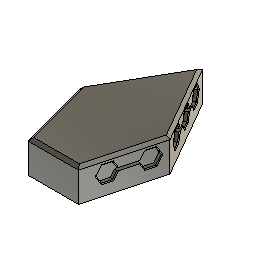
wedge_30deg_0mm (Autodesk Fusion 360 design; units mm, degrees)
Autodesk Fusion 360 part; units mm, degrees
note: some values were not read from the file. Set by a fixed rule: which sketch regions a step uses.
sketch "case_bottom" plane through (0, 0, 0) normal (0, 0, 1) x (1, 0, 0)
  line L0 (-89.0663, -56.676) -> (12.947, -115.5733)
  line L1 (-48.1807, 14.1399) -> (-89.0663, -56.676)
  line L2 (12.947, -115.5733) -> (30.0588, -101.2149)
  line L3 (-25.0151, 15.0605) -> (-48.1807, 14.1399)
  line L4 (11.7937, -0.3589) -> (11.7217, -0.2966)
  line L5 (11.7217, -0.2966) -> (-4.9219, 9.3126)
  line L6 (42.4432, -26.8948) -> (11.7937, -0.3589)
  line L7 (30.0588, -101.2149) -> (20.3625, -65.1396)
  line L8 (20.3625, -65.1396) -> (42.4432, -26.8948)
  line L9 (-4.9219, 9.3126) -> (-25.0151, 15.0605)
  line L10 (-49.952, 17.0719) -> (-93.1644, -57.774)
  line L11 (-93.1644, -57.774) -> (13.2662, -119.2217)
  line L12 (13.4693, 2.1586) -> (-3.7417, 12.0954)
  line L13 (-3.7417, 12.0954) -> (-24.653, 18.0773)
  line L14 (13.2662, -119.2217) -> (33.4524, -102.2834)
  line L15 (23.5826, -65.5623) -> (46.2803, -26.2487)
  line L16 (33.4524, -102.2834) -> (23.5826, -65.5623)
  line L17 (-24.653, 18.0773) -> (-49.952, 17.0719)
  line L18 (46.2803, -26.2487) -> (13.4693, 2.1586)
  line L19 (-4.4498, 10.4257) -> (-24.8703, 16.2672)
  line L20 (-48.8893, 15.3127) -> (-90.7055, -57.1152)
  line L21 (43.9781, -26.6364) -> (12.4207, 0.6855)
  line L22 (13.0747, -117.0327) -> (31.4162, -101.6423)
  line L23 (12.4207, 0.6855) -> (-4.4498, 10.4257)
  line L24 (-24.8703, 16.2672) -> (-48.8893, 15.3127)
  line L25 (31.4162, -101.6423) -> (21.6506, -65.3087)
  line L26 (21.6506, -65.3087) -> (43.9781, -26.6364)
  line L27 (-90.7055, -57.1152) -> (13.0747, -117.0327)
  line L28 (-4.2138, 10.9823) -> (-24.7979, 16.8706)
  line L29 (-91.5252, -57.3348) -> (13.1385, -117.7624)
  line L30 (-49.2435, 15.8991) -> (-91.5252, -57.3348)
  line L31 (12.9719, 1.0019) -> (12.7702, 1.1765)
  line L32 (32.095, -101.856) -> (22.2946, -65.3932)
  line L33 (22.2946, -65.3932) -> (44.7455, -26.5072)
  line L34 (13.1385, -117.7624) -> (32.095, -101.856)
  line L35 (12.7702, 1.1765) -> (-4.2138, 10.9823)
  line L36 (-24.7979, 16.8706) -> (-49.2435, 15.8991)
  line L37 (44.7455, -26.5072) -> (12.9719, 1.0019)
  circle A0 centre (-32.1047, -5.0156) radius 2.2
  circle A1 centre (-51.1047, -37.9246) radius 2.2
  circle A2 centre (12.9286, -31.0156) radius 2.2
  circle A3 centre (4.9904, -77.0362) radius 2.2
  line L38 (-48.2004, -55.8942) -> (-76.7793, -39.3942)
  line L39 (-57.2004, -71.4826) -> (-48.2004, -55.8942)
  line L40 (-85.7793, -54.9826) -> (-57.2004, -71.4826)
  line L41 (-76.7793, -39.3942) -> (-85.7793, -54.9826)
  line L42 (-52.8377, -70.9761) -> (-55.7627, -76.0424)
  line L43 (-48.1417, -80.4424) -> (-45.2167, -75.3761)
  line L44 (-45.2167, -75.3761) -> (-52.8377, -70.9761)
  line L45 (-37.9329, -84.7603) -> (-36.1829, -81.7292)
  line L46 (-43.9771, -77.2292) -> (-45.7271, -80.2603)
  line L47 (-45.7271, -80.2603) -> (-37.9329, -84.7603)
  line L48 (-36.1829, -81.7292) -> (-43.9771, -77.2292)
  line L49 (25.0269, -87.2736) -> (22.1799, -76.6484)
  line L50 (16.237, -89.6289) -> (25.0269, -87.2736)
  line L51 (13.3899, -79.0037) -> (16.237, -89.6289)
  line L52 (22.1799, -76.6484) -> (13.3899, -79.0037)
  line L53 (-49.878, -40.9999) -> (-54.328, -48.7075)
  line L54 (-54.328, -48.7075) -> (-46.8802, -53.0075)
  line L55 (-46.8802, -53.0075) -> (-42.4302, -45.2999)
  line L56 (-42.4302, -45.2999) -> (-49.878, -40.9999)
  line L57 (46.2803, -26.2487) -> (46.2803, -130.4054) construction
  line L58 (178.3399, -54.9826) -> (149.761, -71.4826)
  line L59 (140.7023, -80.4424) -> (137.7773, -75.3761)
  line L60 (70.266, -65.3932) -> (47.8152, -26.5072)
  line L61 (80.7669, -0.3589) -> (80.8389, -0.2966)
  line L62 (145.3983, -70.9761) -> (148.3233, -76.0424)
  circle A4 centre (87.5702, -77.0362) radius 2.2
  line L63 (137.7773, -75.3761) -> (145.3983, -70.9761)
  line L64 (136.5377, -77.2292) -> (138.2877, -80.2603)
  line L65 (128.7435, -81.7292) -> (136.5377, -77.2292)
  line L66 (76.3237, -89.6289) -> (67.5338, -87.2736)
  line L67 (62.5019, -101.2149) -> (72.1981, -65.1396)
  line L68 (79.2945, -119.2217) -> (59.1082, -102.2834)
  line L69 (79.486, -117.0327) -> (61.1444, -101.6423)
  line L70 (70.3808, -76.6484) -> (79.1707, -79.0037)
  line L71 (142.4387, -40.9999) -> (146.8887, -48.7075)
  line L72 (130.4935, -84.7603) -> (128.7435, -81.7292)
  line L73 (67.5338, -87.2736) -> (70.3808, -76.6484)
  line L74 (138.2877, -80.2603) -> (130.4935, -84.7603)
  line L75 (142.5127, 17.0719) -> (185.725, -57.774)
  line L76 (80.1399, 0.6855) -> (97.0105, 10.4257)
  line L77 (48.5826, -26.6364) -> (80.1399, 0.6855)
  line L78 (46.2803, -26.2487) -> (79.0914, 2.1586)
  line L79 (117.2137, 18.0773) -> (142.5127, 17.0719)
  line L80 (79.0914, 2.1586) -> (96.3024, 12.0954)
  line L81 (97.4825, 9.3126) -> (117.5757, 15.0605)
  circle A5 centre (124.6653, -5.0156) radius 2.2
  line L82 (134.9909, -45.2999) -> (142.4387, -40.9999)
  line L83 (169.3399, -39.3942) -> (178.3399, -54.9826)
  line L84 (139.4409, -53.0075) -> (134.9909, -45.2999)
  line L85 (117.3585, 16.8706) -> (141.8041, 15.8991)
  line L86 (146.8887, -48.7075) -> (139.4409, -53.0075)
  line L87 (79.5887, 1.0019) -> (79.7904, 1.1765)
  line L88 (50.1174, -26.8948) -> (80.7669, -0.3589)
  line L89 (149.761, -71.4826) -> (140.761, -55.8942)
  line L90 (184.0858, -57.3348) -> (79.4221, -117.7624)
  line L91 (60.4657, -101.856) -> (70.266, -65.3932)
  line L92 (79.6136, -115.5733) -> (62.5019, -101.2149)
  line L93 (183.2662, -57.1152) -> (79.486, -117.0327)
  line L94 (79.4221, -117.7624) -> (60.4657, -101.856)
  line L95 (47.8152, -26.5072) -> (79.5887, 1.0019)
  line L96 (141.4499, 15.3127) -> (183.2662, -57.1152)
  line L97 (80.8389, -0.2966) -> (97.4825, 9.3126)
  circle A6 centre (143.6653, -37.9246) radius 2.2
  line L98 (140.761, -55.8942) -> (169.3399, -39.3942)
  line L99 (61.1444, -101.6423) -> (70.9101, -65.3087)
  line L100 (59.1082, -102.2834) -> (68.978, -65.5623)
  line L101 (79.1707, -79.0037) -> (76.3237, -89.6289)
  line L102 (185.725, -57.774) -> (79.2945, -119.2217)
  line L103 (181.6269, -56.676) -> (79.6136, -115.5733)
  line L104 (140.7414, 14.1399) -> (181.6269, -56.676)
  line L105 (96.7744, 10.9823) -> (117.3585, 16.8706)
  line L106 (79.7904, 1.1765) -> (96.7744, 10.9823)
  line L107 (96.3024, 12.0954) -> (117.2137, 18.0773)
  line L108 (70.9101, -65.3087) -> (48.5826, -26.6364)
  line L109 (97.0105, 10.4257) -> (117.4309, 16.2672)
  line L110 (117.4309, 16.2672) -> (141.4499, 15.3127)
  line L111 (141.8041, 15.8991) -> (184.0858, -57.3348)
  line L112 (117.5757, 15.0605) -> (140.7414, 14.1399)
  circle A7 centre (79.632, -31.0156) radius 2.2
  line L113 (72.1981, -65.1396) -> (50.1174, -26.8948)
  line L114 (68.978, -65.5623) -> (46.2803, -26.2487)
  line L115 (33.4524, -102.2834) -> (59.1082, -102.2834)
  dimension "d81" = 1.5
  constraint vertical L57
  constraint horizontal L115
extrude "Extrude2" add sketch "case_bottom" along normal blind 16.6 contours L15 L16 L100 L114 L115
sketch "Sketch13" plane through (23.3442, 13.4778, 0) normal (0.866025, 0.5, 0) x (-0.5, 0.866025, 0)
  line L0 (-91.2676, 0) -> (-45.8722, 0)
  line L1 (-45.8722, 0) -> (-45.8722, 16.6)
  line L2 (-45.8722, 16.6) -> (-91.2676, 16.6)
  line L3 (-91.2676, 16.6) -> (-91.2676, 0)
  line L4 (-91.2676, 9.7) -> (-45.8722, 9.7) construction
  line L5 (-79.2676, 13.6708) -> (-83.8576, 13.6792)
  line L6 (-83.8576, 13.6792) -> (-86.1599, 9.7085)
  line L7 (-86.1599, 9.7085) -> (-83.8722, 5.7292)
  line L8 (-83.8722, 5.7292) -> (-79.2823, 5.7208)
  line L9 (-79.2823, 5.7208) -> (-76.98, 9.6915)
  line L10 (-76.98, 9.6915) -> (-79.2676, 13.6708)
  line L11 (-66.2676, 13.6708) -> (-70.8576, 13.6792)
  line L12 (-70.8576, 13.6792) -> (-73.1599, 9.7085)
  line L13 (-73.1599, 9.7085) -> (-70.8722, 5.7292)
  line L14 (-70.8722, 5.7292) -> (-66.2823, 5.7208)
  line L15 (-66.2823, 5.7208) -> (-63.98, 9.6915)
  line L16 (-63.98, 9.6915) -> (-66.2676, 13.6708)
  line L17 (-53.2676, 13.6708) -> (-57.8576, 13.6792)
  line L18 (-57.8576, 13.6792) -> (-60.1599, 9.7085)
  line L19 (-60.1599, 9.7085) -> (-57.8722, 5.7292)
  line L20 (-57.8722, 5.7292) -> (-53.2823, 5.7208)
  line L21 (-53.2823, 5.7208) -> (-50.98, 9.6915)
  line L22 (-50.98, 9.6915) -> (-53.2676, 13.6708)
  line L23 (-81.5699, 8.95) -> (-55.5699, 8.95)
  arc A0 (-55.5699, 8.95) -> (-55.5699, 10.45) centre (-55.5699, 9.7) ccw
  line L24 (-55.5699, 10.45) -> (-81.5699, 10.45)
  arc A1 (-81.5699, 10.45) -> (-81.5699, 8.95) centre (-81.5699, 9.7) ccw
  line L25 (-81.5699, 9.7) -> (-55.5699, 9.7) construction
  point P0 (-68.5699, 9.7)
  point P1 (-81.5699, 9.7)
  point P2 (-55.5699, 9.7)
  point P3 (-81.5699, 9.7)
  point P4 (-68.5699, 9.7)
  point P5 (-55.5699, 9.7)
  dimension "d99" = 6.9
  dimension "d100" = 13
  dimension "d101" = 13
  dimension "d102" = 3.975
  dimension "d103" = 3.975
  dimension "d104" = 3.975
  dimension "d105" = 1.5
  constraint coincident L3 L4.start
  constraint coincident L1 L4.end
  constraint perpendicular L1 L4
  constraint midpoint L4 P4
  constraint coincident L4 P3
  constraint coincident L4 P5
  constraint coincident P3 P1
  constraint coincident P4 P0
  constraint coincident P5 P2
  constraint tangent L23 A0
  constraint tangent A0 L24
  constraint parallel L23 L24
  constraint tangent L24 A1
  constraint tangent L23 A1
  constraint parallel L4 L25
  measures "d99" distance of L2 L4
  measures "d100" distance of P4 P5
  measures "d101" distance of P4 P3
  measures "d102" distance of P3 L10
  measures "d103" distance of P4 L16
  measures "d104" distance of P5 L22
  measures "d105" diameter of A0
extrude "Extrude15" cut sketch "Sketch13" against normal blind 2 contours L5 L6 L7 L8 L9 L10 L23 L24 A1 | L9 L10 L12 L13 L23 L24 | L9 L10 L23 L24 A1 | L12 L13 L15 L16 L23 L24 | L11 L12 L16 L24 | L15 L16 L18 L19 L23 L24 | L13 L14 L15 L23 | L18 L19 L23 A0 L24 | L17 L18 L19 L20 L21 L22 L23 A0 L24
sketch "Sketch14" plane through (46.0763, -26.6022, 0) normal (-0.866025, 0.5, 0) x (-0.5, -0.866025, 0)
  line L0 (-0.4081, 0) -> (44.9873, 0)
  line L1 (44.9873, 0) -> (44.9873, 16.6)
  line L2 (44.9873, 16.6) -> (-0.4081, 16.6)
  line L3 (-0.4081, 16.6) -> (-0.4081, 0)
  line L4 (-0.4081, 9.7) -> (44.9873, 9.7) construction
  line L5 (11.5797, 13.6778) -> (6.9897, 13.6722)
  line L6 (6.9897, 13.6722) -> (4.6997, 9.6943)
  line L7 (4.6997, 9.6943) -> (6.9996, 5.7222)
  line L8 (6.9996, 5.7222) -> (11.5895, 5.7278)
  line L9 (11.5895, 5.7278) -> (13.8795, 9.7057)
  line L10 (13.8795, 9.7057) -> (11.5797, 13.6778)
  line L11 (24.5797, 13.6778) -> (19.9897, 13.6722)
  line L12 (19.9897, 13.6722) -> (17.6997, 9.6943)
  line L13 (17.6997, 9.6943) -> (19.9996, 5.7222)
  line L14 (19.9996, 5.7222) -> (24.5895, 5.7278)
  line L15 (24.5895, 5.7278) -> (26.8795, 9.7057)
  line L16 (26.8795, 9.7057) -> (24.5797, 13.6778)
  line L17 (37.5797, 13.6778) -> (32.9897, 13.6722)
  line L18 (32.9897, 13.6722) -> (30.6997, 9.6943)
  line L19 (30.6997, 9.6943) -> (32.9996, 5.7222)
  line L20 (32.9996, 5.7222) -> (37.5895, 5.7278)
  line L21 (37.5895, 5.7278) -> (39.8795, 9.7057)
  line L22 (39.8795, 9.7057) -> (37.5797, 13.6778)
  line L23 (9.2896, 8.95) -> (35.2896, 8.95)
  arc A0 (35.2896, 8.95) -> (35.2896, 10.45) centre (35.2896, 9.7) ccw
  line L24 (35.2896, 10.45) -> (9.2896, 10.45)
  arc A1 (9.2896, 10.45) -> (9.2896, 8.95) centre (9.2896, 9.7) ccw
  line L25 (9.2896, 9.7) -> (35.2896, 9.7) construction
  point P0 (22.2896, 9.7)
  point P1 (35.2896, 9.7)
  point P2 (9.2896, 9.7)
  point P3 (9.2896, 9.7)
  point P4 (22.2896, 9.7)
  point P5 (35.2896, 9.7)
  dimension "d108" = 6.9
  dimension "d109" = 13
  dimension "d110" = 13
  dimension "d111" = 3.975
  dimension "d112" = 3.975
  dimension "d113" = 3.975
  dimension "d114" = 1.5
  constraint coincident L3 L4.start
  constraint coincident L1 L4.end
  constraint perpendicular L1 L4
  constraint midpoint L4 P4
  constraint coincident L4 P5
  constraint coincident L4 P3
  constraint coincident P3 P2
  constraint coincident P4 P0
  constraint coincident P5 P1
  constraint tangent L23 A0
  constraint tangent A0 L24
  constraint parallel L23 L24
  constraint tangent L24 A1
  constraint tangent L23 A1
  constraint parallel L4 L25
  measures "d108" distance of L2 L4
  measures "d109" distance of P4 P3
  measures "d110" distance of P4 P5
  measures "d111" distance of P3 L10
  measures "d112" distance of P4 L16
  measures "d113" distance of P5 L22
  measures "d114" diameter of A0
extrude "Extrude16" cut sketch "Sketch14" against normal blind 2 contours L5 L6 L7 L8 L9 L10 L23 L24 A1 | L9 L10 L12 L13 L23 L24 | L9 L10 L23 L24 A1 | L12 L13 L15 L16 L23 L24 | L11 L12 L16 L24 | L15 L16 L18 L19 L23 L24 | L13 L14 L15 L23 | L18 L19 L23 A0 L24 | L17 L18 L19 L20 L21 L22 L23 A0 L24
sketch "Sketch15" plane through (5.5593, 1.4942, 0) normal (-0.965726, -0.259565, 0) x (0.259565, -0.965726, 0)
  line L0 (69.4364, 0) -> (107.4608, 0)
  line L1 (107.4608, 0) -> (107.4608, 16.6)
  line L2 (107.4608, 16.6) -> (69.4364, 16.6)
  line L3 (69.4364, 16.6) -> (69.4364, 0)
  line L4 (69.4364, 9.7) -> (107.4608, 9.7) construction
  line L5 (79.7376, 13.6714) -> (75.1477, 13.6786)
  line L6 (75.1477, 13.6786) -> (72.8465, 9.7072)
  line L7 (72.8465, 9.7072) -> (75.1352, 5.7286)
  line L8 (75.1352, 5.7286) -> (79.7251, 5.7214)
  line L9 (79.7251, 5.7214) -> (82.0264, 9.6928)
  line L10 (82.0264, 9.6928) -> (79.7376, 13.6714)
  line L11 (90.8709, 9.6928) -> (93.1721, 5.7214)
  line L12 (93.1721, 5.7214) -> (97.762, 5.7286)
  line L13 (97.762, 5.7286) -> (100.0508, 9.7072)
  line L14 (100.0508, 9.7072) -> (97.7495, 13.6786)
  line L15 (97.7495, 13.6786) -> (93.1596, 13.6714)
  line L16 (93.1596, 13.6714) -> (90.8709, 9.6928)
  line L17 (77.4364, 8.95) -> (95.4608, 8.95)
  arc A0 (95.4608, 8.95) -> (95.4608, 10.45) centre (95.4608, 9.7) ccw
  line L18 (95.4608, 10.45) -> (77.4364, 10.45)
  arc A1 (77.4364, 10.45) -> (77.4364, 8.95) centre (77.4364, 9.7) ccw
  line L19 (77.4364, 9.7) -> (95.4608, 9.7) construction
  point P0 (77.4364, 9.7)
  point P1 (95.4608, 9.7)
  point P2 (77.4364, 9.7)
  point P3 (95.4608, 9.7)
  dimension "d117" = 6.9
  dimension "d118" = 8
  dimension "d119" = 12
  dimension "d120" = 3.975
  dimension "d121" = 3.975
  dimension "d122" = 1.5
  constraint coincident L3 L4.start
  constraint coincident L1 L4.end
  constraint perpendicular L1 L4
  constraint coincident L4 P2
  constraint coincident L4 P3
  constraint coincident P2 P0
  constraint coincident P3 P1
  constraint tangent L17 A0
  constraint tangent A0 L18
  constraint parallel L17 L18
  constraint tangent L18 A1
  constraint tangent L17 A1
  constraint parallel L4 L19
  measures "d117" distance of L2 L4
  measures "d118" distance of L3 P2
  measures "d119" distance of L1 P3
  measures "d120" distance of P2 L10
  measures "d121" distance of P3 L16
  measures "d122" diameter of A0
extrude "Extrude17" cut sketch "Sketch15" against normal blind 2 contours L5 L6 L7 L8 L9 L10 L17 L18 A1 | L9 L10 L11 L16 L17 L18 | L9 L10 L17 L18 A1 | L11 L16 L17 A0 L18 | L11 L12 L13 L14 L15 L16 L17 A0 L18
sketch "Sketch16" plane through (80.7651, -21.7078, 0) normal (0.965726, -0.259565, 0) x (0.259565, 0.965726, 0)
  line L0 (-83.4353, 0) -> (-45.4109, 0)
  line L1 (-45.4109, 0) -> (-45.4109, 16.6)
  line L2 (-45.4109, 16.6) -> (-83.4353, 16.6)
  line L3 (-83.4353, 16.6) -> (-83.4353, 0)
  line L4 (-83.4353, 9.7) -> (-45.4109, 9.7) construction
  line L5 (-69.1608, 13.6868) -> (-73.7507, 13.6631)
  line L6 (-73.7507, 13.6631) -> (-76.0252, 9.6764)
  line L7 (-76.0252, 9.6764) -> (-73.7098, 5.7132)
  line L8 (-73.7098, 5.7132) -> (-69.1199, 5.7369)
  line L9 (-69.1199, 5.7369) -> (-66.8454, 9.7236)
  line L10 (-66.8454, 9.7236) -> (-69.1608, 13.6868)
  line L11 (-58.0008, 9.7236) -> (-55.7263, 5.7369)
  line L12 (-55.7263, 5.7369) -> (-51.1364, 5.7132)
  line L13 (-51.1364, 5.7132) -> (-48.821, 9.6764)
  line L14 (-48.821, 9.6764) -> (-51.0955, 13.6631)
  line L15 (-51.0955, 13.6631) -> (-55.6854, 13.6868)
  line L16 (-55.6854, 13.6868) -> (-58.0008, 9.7236)
  line L17 (-53.4109, 10.45) -> (-71.4353, 10.45)
  arc A0 (-71.4353, 10.45) -> (-71.4353, 8.95) centre (-71.4353, 9.7) ccw
  line L18 (-71.4353, 8.95) -> (-53.4109, 8.95)
  arc A1 (-53.4109, 8.95) -> (-53.4109, 10.45) centre (-53.4109, 9.7) ccw
  line L19 (-53.4109, 9.7) -> (-71.4353, 9.7) construction
  point P0 (-71.4353, 9.7)
  point P1 (-53.4109, 9.7)
  point P2 (-71.4353, 9.7)
  point P3 (-53.4109, 9.7)
  dimension "d125" = 6.9
  dimension "d126" = 8
  dimension "d127" = 12
  dimension "d128" = 3.975
  dimension "d129" = 3.975
  dimension "d130" = 1.5
  constraint coincident L3 L4.start
  constraint coincident L1 L4.end
  constraint perpendicular L1 L4
  constraint coincident L4 P2
  constraint coincident L4 P3
  constraint coincident P2 P0
  constraint coincident P3 P1
  constraint tangent L17 A0
  constraint tangent A0 L18
  constraint parallel L17 L18
  constraint tangent L18 A1
  constraint tangent L17 A1
  constraint parallel L4 L19
  measures "d125" distance of L2 L4
  measures "d126" distance of L1 P3
  measures "d127" distance of L3 P2
  measures "d128" distance of P2 L10
  measures "d129" distance of P3 L16
  measures "d130" diameter of A0
extrude "Extrude18" cut sketch "Sketch16" against normal blind 2 contours L5 L6 L7 L8 L9 L10 L17 A0 L18 | L9 L10 L11 L16 L17 L18 | L9 L10 L17 A0 L18 | L11 L16 L17 L18 A1 | L11 L12 L13 L14 L15 L16 L17 L18 A1
chamfer "Chamfer4" distance 0.4 angle 45 60 edges at (43.1539, -31.6638, 11.6832) (41.4339, -34.6429, 13.675) (43.1515, -31.6681, 7.7082) (41.429, -34.6514, 5.725) (39.8178, -37.4422, 7.3389) (39.8192, -37.4397, 12.0639) (36.5452, -43.1105, 12.0611) (34.9339, -45.9013, 13.675) (33.3192, -48.698, 12.0639) (36.5437, -43.113, 7.3361) (34.929, -45.9098, 5.725) (33.3178, -48.7005, 7.3389) (30.0452, -54.3689, 12.0611) (28.4339, -57.1596, 13.675) (26.7115, -60.143, 11.6918) (26.709, -60.1472, 7.7168) (28.429, -57.1681, 5.725) (30.0437, -54.3713, 7.3361) (24.7664, -69.9667, 11.6929) (25.6608, -73.2942, 13.675) (26.497, -76.4053, 12.0607) (24.7648, -69.9606, 7.7179) (25.6575, -73.2821, 5.725) (26.496, -76.4017, 7.3357) (29.4998, -87.5776, 12.0607) (30.336, -90.6887, 13.675) (29.5008, -87.5811, 7.3357) (30.3393, -90.7008, 5.725) (31.232, -94.0222, 7.7179) (31.2304, -94.0162, 11.6929) (62.2177, -90.7145, 13.6749) (61.3268, -94.029, 11.6697) (61.3321, -94.0093, 7.6948) (62.2283, -90.675, 5.7251) (63.0619, -87.5736, 7.3434) (63.0588, -87.5851, 12.0684) (66.0657, -76.3977, 12.0684) (66.9068, -73.2683, 13.6749) (66.0626, -76.4093, 7.3434) (66.8962, -73.3079, 5.7251) (67.7924, -69.9736, 7.6948) (67.7977, -69.9538, 11.6697) (65.8486, -60.1419, 11.6939) (65.8522, -60.1483, 7.7189) (64.1255, -57.1575, 13.675) (62.5151, -54.3682, 12.0604) (64.1328, -57.1702, 5.725) (62.5173, -54.372, 7.3354) (59.2411, -48.6974, 12.0646) (59.2432, -48.7011, 7.3396) (57.6328, -45.9119, 5.725) (56.0173, -43.1136, 7.3354) (56.0151, -43.1099, 12.0604) (57.6255, -45.8992, 13.675) (52.7411, -37.4391, 12.0646) (51.1255, -34.6408, 13.675) (52.7432, -37.4428, 7.3396) (51.1328, -34.6536, 5.725) (49.4098, -31.6691, 7.7061) (49.4061, -31.6628, 11.6811)
chamfer "Chamfer5" distance 1.5 angle 45 1 faces at (46.2803, -52.4578, 16.6)
equation "rotation = 15 deg"
equation "mirror_offset = 2 mm"
